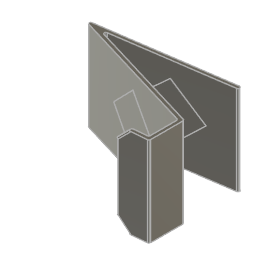
Nook Tablet Stand (Autodesk Fusion 360 design; units mm, degrees)
Autodesk Fusion 360 part; units mm, degrees
sketch "Sketch1" plane through (0, 0, 0) normal (1, 0, 0) x (0, 1, 0)
  line L0 (0, 0) -> (60, 200) construction
  line L1 (-41.0372, 13.6) -> (-39.9873, 1.6)
  line L2 (-39.9873, 1.6) -> (-26.9873, 1.6)
  line L3 (-26.9873, 1.6) -> (-8.9873, 61.6)
  line L4 (-8.9873, 61.6) -> (-0.2334, 1.6)
  line L5 (-42.6311, 13.4606) -> (-41.4534, 0)
  line L6 (-41.4534, 0) -> (-25.7968, 0)
  line L7 (-25.7968, 0) -> (-9.5286, 54.2275)
  line L8 (-9.5286, 54.2275) -> (-1.6169, 0)
  line L9 (-0.2334, 1.6) -> (0, 0)
  line L10 (-1.6169, 0) -> (0, 0)
  line L11 (-41.0372, 13.6) -> (-42.6311, 13.4606)
  dimension "d1" = 60
  dimension "d2" = 200
  dimension "d3" = 60
  dimension "d4" = 13
  dimension "d5" = 12
  dimension "d6" = 95
  dimension "d7" = 25
  dimension "d8" = 1.6
  constraint coincident L0.start L9.end
  constraint horizontal L2
  constraint parallel L0 L3
  constraint coincident L2 L4.end
  constraint parallel L4 L9
  constraint collinear L6 L10
  constraint perpendicular L5 L11
  measures "d1" horizontal distance of L0.start L0.end
  measures "d2" vertical distance of L0.start L0.end
  measures "d3" vertical distance of L2.end L3.end
  measures "d4" distance of L1.end L2.end
  measures "d5" vertical distance of L1.start L1.end
  measures "d6" angle of L1 L2
  measures "d7" angle of L3 L4
extrude "Extrude1" add sketch "Sketch1" along normal mid plane 40 makes body 1
chamfer "Chamfer1" distance 5 angle 45 2 edges at (-20, -41.8341, 13.5303) (20, -41.8341, 13.5303) on bodies 1
fillet "Fillet1" radius 0.7 14 edges at (0, -42.6311, 13.4606) (0, -41.0372, 13.6) (0, -41.4534, 0) (0, -26.9873, 1.6) (0, -39.9873, 1.6) (0, -25.7968, 0) (0, -1.6169, 0) (0, 0, 0) (0, -9.5286, 54.2275) (0, -8.9873, 61.6) (-17.5, -42.4132, 10.9701) (-17.5, -40.8193, 11.1095) (17.5, -42.4132, 10.9701) (17.5, -40.8193, 11.1095) on bodies 1
move_body "Move1" bodies 1 to x (0, 0, 1) y (0, 1, 0) z (-1, 0, 0) at (-20, 0, 20)
sketch "Sketch2" plane through (-9.2112, -30.7039, 0) normal (-0.287348, -0.957826, 0) x (0.957826, -0.287348, 0)
  line L0 (-72.4186, 40) -> (-72.4186, 0)
  line L1 (-72.4186, 0) -> (-13.4551, 0)
  line L2 (-13.4551, 0) -> (-13.4551, 40)
  line L3 (-13.4551, 40) -> (-72.4186, 40)
  line L4 (-65.2015, 0) -> (-12.2647, 0)
  line L5 (-65.2015, 0) -> (-65.2015, 7.2171) construction
  line L6 (-13.4551, 40) -> (-13.4551, 0)
  line L7 (-20.6723, 7.2171) -> (-65.2015, 7.2171) construction
  line L8 (-72.4186, 20) -> (-64.2336, 20) construction
  line L9 (-20.6723, 32.7829) -> (-65.2015, 32.7829) construction
  line L10 (-65.2015, 32.7829) -> (-65.2015, 7.2171)
  line L11 (-20.6723, 32.7829) -> (-20.6723, 7.2171)
  line L12 (-42.9369, 7.2171) -> (-30.1583, 20.3313)
  line L13 (-30.1583, 20.3313) -> (-42.9369, 32.7829)
  line L14 (-42.9369, 7.2171) -> (-55.7155, 20.3313)
  line L15 (-55.7155, 20.3313) -> (-42.9369, 32.7829)
  dimension "d14" = 7.2171
  dimension "d15" = 7.2171
  dimension "d16" = 7.2171
  constraint coincident L4.start L5.start
  constraint perpendicular L4 L5
  constraint perpendicular L5 L7
  constraint midpoint L0 L8.start
  constraint perpendicular L0 L8
  constraint symmetric L5.end L8 L9.end
  constraint symmetric L7.start L8 L9.start
  constraint coincident L7 L12.start
  constraint midpoint L9 L13.end
  constraint vertical L12.start L13.end
  constraint equal L13 L15
  constraint equal L12 L14
  constraint perpendicular L14 L15
  measures "d14" distance of L0 L5
  measures "d15" distance of L2 L7.start
  measures "d16" distance of L4.start L5.end
split "Split1" by curves path "Sketch2" along L13 L12 L14 L15 bodies 1 makes body 2 at (-50.3373, -18.3661, 15.9599) makes body 3 at (-27.4318, -25.2378, 20.1104)
equation "d15 = d14"
equation "d16 = d14"
